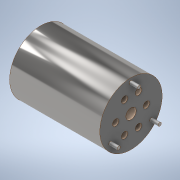
# Autodesk Inventor part: DC SUBMERSIBLE PUMP
Saved by Autodesk Inventor 2021 (Build 250183000, 183)
## iProperties
Created: 2021-07-11
Part Number: DC SUBMERSIBLE PUMP
Material: Generic
Document SubType Name: Modeling
Designer: HP
Density: 1 g/cm^3
Appearance: Exterior - Beige
Author: HP
Autodesk Inventor part; units mm, degrees
ref_plane "YZ Plane" through (0, 0, 0) normal (1, 0, 0) x (0, 1, 0)
ref_plane "XZ Plane" through (0, 0, 0) normal (0, 1, 0) x (-1, 0, 0)
ref_plane "XY Plane" through (0, 0, 0) normal (0, 0, 1) x (1, 0, 0)
sketch "Sketch1" plane through (0, 0, 0) normal (1, 0, 0) x (0, 1, 0)
  circle A0 centre (0, 0) radius 9.6564
  constraints: 1 centre point
extrude "Extrusion1" add sketch "Sketch1" along normal blind 15.24
sketch "Sketch2" plane through (15.24, 0, 0) normal (1, 0, 0) x (0, 0, -1)
  circle A0 centre (0, 0) radius 6.5454
  circle A1 centre (0, 0) radius 1.5875
  circle A2 centre (-4.7625, 0) radius 0.9525
  circle A3 centre (2.3204, 4.7625) radius 0.9525
  circle A4 centre (4.7625, 0) radius 0.9525
  circle A5 centre (2.3204, -4.7625) radius 0.9525
  circle A6 centre (-2.0084, -4.7625) radius 0.9525
  circle A7 centre (-2.0084, 4.7625) radius 0.9525
  circle A8 centre (0, 8.2286) radius 0.508
  circle A9 centre (-5.715, -5.715) radius 0.508
  circle A10 centre (5.715, -5.715) radius 0.508
  dimension "d3" = 1.905
  dimension "d5" = 1.905
  dimension "d6" = 1.905
  dimension "d7" = 1.905
  dimension "d8" = 1.905
  dimension "d9" = 1.905
  dimension "d10" = 1.016
  dimension "d11" = 1.016
  dimension "d12" = 1.016
  constraints: 11 centre point, 2 coincident
  measures "d3" diameter of A2
  measures "d5" diameter of A3
  measures "d6" diameter of A4
  measures "d7" diameter of A5
  measures "d8" diameter of A6
  measures "d9" diameter of A7
  measures "d10" diameter of A8
  measures "d11" diameter of A9
  measures "d12" diameter of A10
extrude "Extrusion2" cut sketch "Sketch2" against normal blind 10.16 contours A1 | A2 | A3 | A4 | A5 | A6 | A7
sketch "Sketch3" plane through (15.24, 0, 0) normal (1, 0, 0) x (0, 0, -1)
  circle A0 centre (0, 8.3846) radius 0.508
  circle A1 centre (-6.35, -4.7625) radius 0.508
  circle A2 centre (6.35, -4.7625) radius 0.508
  point P0 (0, 0)
  dimension "d15" = 1.016
  dimension "d16" = 1.016
  dimension "d17" = 1.016
  constraints: 3 centre point
  measures "d15" diameter of A0
  measures "d16" diameter of A1
  measures "d17" diameter of A2
extrude "Extrusion3" add sketch "Sketch3" along normal blind 2.54
sketch "Sketch4" plane through (0, 0, 0) normal (-1, 0, 0) x (0, 0, 1)
  circle A0 centre (0, 0) radius 9.6564
  constraints: 1 centre point, 1 coincident
extrude "Extrusion4" add sketch "Sketch4" along normal blind 12.7
body "Solid1"
